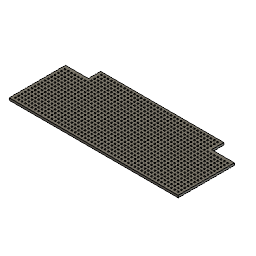
trunk mounting plate (Autodesk Fusion 360 design; units mm, degrees)
Autodesk Fusion 360 part; units mm, degrees
(part 1 of 2)
sketch "Sketch1" plane through (0, 0, 0) normal (0, 1, 0) x (1, 0, 0)
  line L0 (480, -195) -> (0, -195)
  line L1 (415, 0) -> (415, -35)
  line L2 (415, -35) -> (480, -35)
  line L3 (65, 0) -> (65, -35)
  line L4 (65, -35) -> (0, -35)
  line L5 (0, -195) -> (0, -35)
  line L6 (65, 0) -> (415, 0)
  line L7 (480, -35) -> (480, -195)
  circle A0 centre (9, -186) radius 2.25
  circle A1 centre (18.4286, -186) radius 2.25
  circle A2 centre (27.8571, -186) radius 2.25
  circle A3 centre (37.2857, -186) radius 2.25
  circle A4 centre (46.7143, -186) radius 2.25
  circle A5 centre (56.1429, -186) radius 2.25
  circle A6 centre (65.5714, -186) radius 2.25
  circle A7 centre (75, -186) radius 2.25
  circle A8 centre (84.4286, -186) radius 2.25
  circle A9 centre (93.8571, -186) radius 2.25
  circle A10 centre (103.2857, -186) radius 2.25
  circle A11 centre (112.7143, -186) radius 2.25
  circle A12 centre (122.1429, -186) radius 2.25
  circle A13 centre (131.5714, -186) radius 2.25
  circle A14 centre (141, -186) radius 2.25
  circle A15 centre (150.4286, -186) radius 2.25
  circle A16 centre (159.8571, -186) radius 2.25
  circle A17 centre (169.2857, -186) radius 2.25
  circle A18 centre (178.7143, -186) radius 2.25
  circle A19 centre (188.1429, -186) radius 2.25
  circle A20 centre (197.5714, -186) radius 2.25
  circle A21 centre (207, -186) radius 2.25
  circle A22 centre (216.4286, -186) radius 2.25
  circle A23 centre (225.8571, -186) radius 2.25
  circle A24 centre (235.2857, -186) radius 2.25
  circle A25 centre (244.7143, -186) radius 2.25
  circle A26 centre (254.1429, -186) radius 2.25
  circle A27 centre (263.5714, -186) radius 2.25
  circle A28 centre (273, -186) radius 2.25
  circle A29 centre (282.4286, -186) radius 2.25
  circle A30 centre (291.8571, -186) radius 2.25
  circle A31 centre (301.2857, -186) radius 2.25
  circle A32 centre (310.7143, -186) radius 2.25
  circle A33 centre (320.1429, -186) radius 2.25
  circle A34 centre (329.5714, -186) radius 2.25
  circle A35 centre (339, -186) radius 2.25
  circle A36 centre (348.4286, -186) radius 2.25
  circle A37 centre (357.8571, -186) radius 2.25
  circle A38 centre (367.2857, -186) radius 2.25
  circle A39 centre (376.7143, -186) radius 2.25
  circle A40 centre (386.1429, -186) radius 2.25
  circle A41 centre (395.5714, -186) radius 2.25
  circle A42 centre (405, -186) radius 2.25
  circle A43 centre (414.4286, -186) radius 2.25
  circle A44 centre (423.8571, -186) radius 2.25
  circle A45 centre (433.2857, -186) radius 2.25
  circle A46 centre (442.7143, -186) radius 2.25
  circle A47 centre (452.1429, -186) radius 2.25
  circle A48 centre (461.5714, -186) radius 2.25
  circle A49 centre (471, -186) radius 2.25
  circle A50 centre (9, -176.6421) radius 2.25
  circle A51 centre (18.4286, -176.6421) radius 2.25
  circle A52 centre (27.8571, -176.6421) radius 2.25
  circle A53 centre (37.2857, -176.6421) radius 2.25
  circle A54 centre (46.7143, -176.6421) radius 2.25
  circle A55 centre (56.1429, -176.6421) radius 2.25
  circle A56 centre (65.5714, -176.6421) radius 2.25
  circle A57 centre (75, -176.6421) radius 2.25
  circle A58 centre (84.4286, -176.6421) radius 2.25
  circle A59 centre (93.8571, -176.6421) radius 2.25
  circle A60 centre (103.2857, -176.6421) radius 2.25
  circle A61 centre (112.7143, -176.6421) radius 2.25
  circle A62 centre (122.1429, -176.6421) radius 2.25
  circle A63 centre (131.5714, -176.6421) radius 2.25
  circle A64 centre (141, -176.6421) radius 2.25
  circle A65 centre (150.4286, -176.6421) radius 2.25
  circle A66 centre (159.8571, -176.6421) radius 2.25
  circle A67 centre (169.2857, -176.6421) radius 2.25
  circle A68 centre (178.7143, -176.6421) radius 2.25
  circle A69 centre (188.1429, -176.6421) radius 2.25
  circle A70 centre (197.5714, -176.6421) radius 2.25
  circle A71 centre (207, -176.6421) radius 2.25
  circle A72 centre (216.4286, -176.6421) radius 2.25
  circle A73 centre (225.8571, -176.6421) radius 2.25
  circle A74 centre (235.2857, -176.6421) radius 2.25
  circle A75 centre (244.7143, -176.6421) radius 2.25
  circle A76 centre (254.1429, -176.6421) radius 2.25
  circle A77 centre (263.5714, -176.6421) radius 2.25
  circle A78 centre (273, -176.6421) radius 2.25
  circle A79 centre (282.4286, -176.6421) radius 2.25
  circle A80 centre (291.8571, -176.6421) radius 2.25
  circle A81 centre (301.2857, -176.6421) radius 2.25
  circle A82 centre (310.7143, -176.6421) radius 2.25
  circle A83 centre (320.1429, -176.6421) radius 2.25
  circle A84 centre (329.5714, -176.6421) radius 2.25
  circle A85 centre (339, -176.6421) radius 2.25
  circle A86 centre (348.4286, -176.6421) radius 2.25
  circle A87 centre (357.8571, -176.6421) radius 2.25
  circle A88 centre (367.2857, -176.6421) radius 2.25
  circle A89 centre (376.7143, -176.6421) radius 2.25
  circle A90 centre (386.1429, -176.6421) radius 2.25
  circle A91 centre (395.5714, -176.6421) radius 2.25
  circle A92 centre (405, -176.6421) radius 2.25
  circle A93 centre (414.4286, -176.6421) radius 2.25
  circle A94 centre (423.8571, -176.6421) radius 2.25
  circle A95 centre (433.2857, -176.6421) radius 2.25
  circle A96 centre (442.7143, -176.6421) radius 2.25
  circle A97 centre (452.1429, -176.6421) radius 2.25
  circle A98 centre (461.5714, -176.6421) radius 2.25
  circle A99 centre (471, -176.6421) radius 2.25
  circle A100 centre (9, -167.2842) radius 2.25
  circle A101 centre (18.4286, -167.2842) radius 2.25
  circle A102 centre (27.8571, -167.2842) radius 2.25
  circle A103 centre (37.2857, -167.2842) radius 2.25
  circle A104 centre (46.7143, -167.2842) radius 2.25
  circle A105 centre (56.1429, -167.2842) radius 2.25
  circle A106 centre (65.5714, -167.2842) radius 2.25
  circle A107 centre (75, -167.2842) radius 2.25
  circle A108 centre (84.4286, -167.2842) radius 2.25
  circle A109 centre (93.8571, -167.2842) radius 2.25
  circle A110 centre (103.2857, -167.2842) radius 2.25
  circle A111 centre (112.7143, -167.2842) radius 2.25
  circle A112 centre (122.1429, -167.2842) radius 2.25
  circle A113 centre (131.5714, -167.2842) radius 2.25
  circle A114 centre (141, -167.2842) radius 2.25
  circle A115 centre (150.4286, -167.2842) radius 2.25
  circle A116 centre (159.8571, -167.2842) radius 2.25
  circle A117 centre (169.2857, -167.2842) radius 2.25
  circle A118 centre (178.7143, -167.2842) radius 2.25
  circle A119 centre (188.1429, -167.2842) radius 2.25
  circle A120 centre (197.5714, -167.2842) radius 2.25
  circle A121 centre (207, -167.2842) radius 2.25
  circle A122 centre (216.4286, -167.2842) radius 2.25
  circle A123 centre (225.8571, -167.2842) radius 2.25
  circle A124 centre (235.2857, -167.2842) radius 2.25
  circle A125 centre (244.7143, -167.2842) radius 2.25
  circle A126 centre (254.1429, -167.2842) radius 2.25
  circle A127 centre (263.5714, -167.2842) radius 2.25
  circle A128 centre (273, -167.2842) radius 2.25
  circle A129 centre (282.4286, -167.2842) radius 2.25
  circle A130 centre (291.8571, -167.2842) radius 2.25
  circle A131 centre (301.2857, -167.2842) radius 2.25
  circle A132 centre (310.7143, -167.2842) radius 2.25
  circle A133 centre (320.1429, -167.2842) radius 2.25
  circle A134 centre (329.5714, -167.2842) radius 2.25
  circle A135 centre (339, -167.2842) radius 2.25
  circle A136 centre (348.4286, -167.2842) radius 2.25
  circle A137 centre (357.8571, -167.2842) radius 2.25
  circle A138 centre (367.2857, -167.2842) radius 2.25
  circle A139 centre (376.7143, -167.2842) radius 2.25
  circle A140 centre (386.1429, -167.2842) radius 2.25
  circle A141 centre (395.5714, -167.2842) radius 2.25
  circle A142 centre (405, -167.2842) radius 2.25
  circle A143 centre (414.4286, -167.2842) radius 2.25
  circle A144 centre (423.8571, -167.2842) radius 2.25
  circle A145 centre (433.2857, -167.2842) radius 2.25
  circle A146 centre (442.7143, -167.2842) radius 2.25
  circle A147 centre (452.1429, -167.2842) radius 2.25
  circle A148 centre (461.5714, -167.2842) radius 2.25
  circle A149 centre (471, -167.2842) radius 2.25
  circle A150 centre (9, -157.9263) radius 2.25
  circle A151 centre (18.4286, -157.9263) radius 2.25
  circle A152 centre (27.8571, -157.9263) radius 2.25
  circle A153 centre (37.2857, -157.9263) radius 2.25
  circle A154 centre (46.7143, -157.9263) radius 2.25
  circle A155 centre (56.1429, -157.9263) radius 2.25
  circle A156 centre (65.5714, -157.9263) radius 2.25
  circle A157 centre (75, -157.9263) radius 2.25
  circle A158 centre (84.4286, -157.9263) radius 2.25
  circle A159 centre (93.8571, -157.9263) radius 2.25
  circle A160 centre (103.2857, -157.9263) radius 2.25
  circle A161 centre (112.7143, -157.9263) radius 2.25
  circle A162 centre (122.1429, -157.9263) radius 2.25
  circle A163 centre (131.5714, -157.9263) radius 2.25
  circle A164 centre (141, -157.9263) radius 2.25
  circle A165 centre (150.4286, -157.9263) radius 2.25
  circle A166 centre (159.8571, -157.9263) radius 2.25
  circle A167 centre (169.2857, -157.9263) radius 2.25
  circle A168 centre (178.7143, -157.9263) radius 2.25
  circle A169 centre (188.1429, -157.9263) radius 2.25
  circle A170 centre (197.5714, -157.9263) radius 2.25
  circle A171 centre (207, -157.9263) radius 2.25
  circle A172 centre (216.4286, -157.9263) radius 2.25
  circle A173 centre (225.8571, -157.9263) radius 2.25
  circle A174 centre (235.2857, -157.9263) radius 2.25
  circle A175 centre (244.7143, -157.9263) radius 2.25
  circle A176 centre (254.1429, -157.9263) radius 2.25
  circle A177 centre (263.5714, -157.9263) radius 2.25
  circle A178 centre (273, -157.9263) radius 2.25
  circle A179 centre (282.4286, -157.9263) radius 2.25
  circle A180 centre (291.8571, -157.9263) radius 2.25
  circle A181 centre (301.2857, -157.9263) radius 2.25
  circle A182 centre (310.7143, -157.9263) radius 2.25
  circle A183 centre (320.1429, -157.9263) radius 2.25
  circle A184 centre (329.5714, -157.9263) radius 2.25
  circle A185 centre (339, -157.9263) radius 2.25
  circle A186 centre (348.4286, -157.9263) radius 2.25
  circle A187 centre (357.8571, -157.9263) radius 2.25
  circle A188 centre (367.2857, -157.9263) radius 2.25
  circle A189 centre (376.7143, -157.9263) radius 2.25
  circle A190 centre (386.1429, -157.9263) radius 2.25
  circle A191 centre (395.5714, -157.9263) radius 2.25
  circle A192 centre (405, -157.9263) radius 2.25
  circle A193 centre (414.4286, -157.9263) radius 2.25
  circle A194 centre (423.8571, -157.9263) radius 2.25
  circle A195 centre (433.2857, -157.9263) radius 2.25
  circle A196 centre (442.7143, -157.9263) radius 2.25
  circle A197 centre (452.1429, -157.9263) radius 2.25
  circle A198 centre (461.5714, -157.9263) radius 2.25
  circle A199 centre (471, -157.9263) radius 2.25
  circle A200 centre (9, -148.5684) radius 2.25
  circle A201 centre (18.4286, -148.5684) radius 2.25
  circle A202 centre (27.8571, -148.5684) radius 2.25
  circle A203 centre (37.2857, -148.5684) radius 2.25
  circle A204 centre (46.7143, -148.5684) radius 2.25
  circle A205 centre (56.1429, -148.5684) radius 2.25
  circle A206 centre (65.5714, -148.5684) radius 2.25
  circle A207 centre (75, -148.5684) radius 2.25
  circle A208 centre (84.4286, -148.5684) radius 2.25
  circle A209 centre (93.8571, -148.5684) radius 2.25
  circle A210 centre (103.2857, -148.5684) radius 2.25
  circle A211 centre (112.7143, -148.5684) radius 2.25
  circle A212 centre (122.1429, -148.5684) radius 2.25
  circle A213 centre (131.5714, -148.5684) radius 2.25
  circle A214 centre (141, -148.5684) radius 2.25
  circle A215 centre (150.4286, -148.5684) radius 2.25
  circle A216 centre (159.8571, -148.5684) radius 2.25
  circle A217 centre (169.2857, -148.5684) radius 2.25
  circle A218 centre (178.7143, -148.5684) radius 2.25
  circle A219 centre (188.1429, -148.5684) radius 2.25
  circle A220 centre (197.5714, -148.5684) radius 2.25
  circle A221 centre (207, -148.5684) radius 2.25
  circle A222 centre (216.4286, -148.5684) radius 2.25
  circle A223 centre (225.8571, -148.5684) radius 2.25
  circle A224 centre (235.2857, -148.5684) radius 2.25
  circle A225 centre (244.7143, -148.5684) radius 2.25
  circle A226 centre (254.1429, -148.5684) radius 2.25
  circle A227 centre (263.5714, -148.5684) radius 2.25
  circle A228 centre (273, -148.5684) radius 2.25
  circle A229 centre (282.4286, -148.5684) radius 2.25
  circle A230 centre (291.8571, -148.5684) radius 2.25
  circle A231 centre (301.2857, -148.5684) radius 2.25
  circle A232 centre (310.7143, -148.5684) radius 2.25
  circle A233 centre (320.1429, -148.5684) radius 2.25
  circle A234 centre (329.5714, -148.5684) radius 2.25
  circle A235 centre (339, -148.5684) radius 2.25
  circle A236 centre (348.4286, -148.5684) radius 2.25
  circle A237 centre (357.8571, -148.5684) radius 2.25
  circle A238 centre (367.2857, -148.5684) radius 2.25
  circle A239 centre (376.7143, -148.5684) radius 2.25
  circle A240 centre (386.1429, -148.5684) radius 2.25
  circle A241 centre (395.5714, -148.5684) radius 2.25
  circle A242 centre (405, -148.5684) radius 2.25
  circle A243 centre (414.4286, -148.5684) radius 2.25
  circle A244 centre (423.8571, -148.5684) radius 2.25
  circle A245 centre (433.2857, -148.5684) radius 2.25
  circle A246 centre (442.7143, -148.5684) radius 2.25
  circle A247 centre (452.1429, -148.5684) radius 2.25
  circle A248 centre (461.5714, -148.5684) radius 2.25
  circle A249 centre (471, -148.5684) radius 2.25
  circle A250 centre (9, -139.2105) radius 2.25
  circle A251 centre (18.4286, -139.2105) radius 2.25
  circle A252 centre (27.8571, -139.2105) radius 2.25
  circle A253 centre (37.2857, -139.2105) radius 2.25
  circle A254 centre (46.7143, -139.2105) radius 2.25
  circle A255 centre (56.1429, -139.2105) radius 2.25
  circle A256 centre (65.5714, -139.2105) radius 2.25
  circle A257 centre (75, -139.2105) radius 2.25
  circle A258 centre (84.4286, -139.2105) radius 2.25
  circle A259 centre (93.8571, -139.2105) radius 2.25
  circle A260 centre (103.2857, -139.2105) radius 2.25
  circle A261 centre (112.7143, -139.2105) radius 2.25
  circle A262 centre (122.1429, -139.2105) radius 2.25
  circle A263 centre (131.5714, -139.2105) radius 2.25
  circle A264 centre (141, -139.2105) radius 2.25
  circle A265 centre (150.4286, -139.2105) radius 2.25
  circle A266 centre (159.8571, -139.2105) radius 2.25
  circle A267 centre (169.2857, -139.2105) radius 2.25
  circle A268 centre (178.7143, -139.2105) radius 2.25
  circle A269 centre (188.1429, -139.2105) radius 2.25
  circle A270 centre (197.5714, -139.2105) radius 2.25
  circle A271 centre (207, -139.2105) radius 2.25
  circle A272 centre (216.4286, -139.2105) radius 2.25
  circle A273 centre (225.8571, -139.2105) radius 2.25
  circle A274 centre (235.2857, -139.2105) radius 2.25
  circle A275 centre (244.7143, -139.2105) radius 2.25
  circle A276 centre (254.1429, -139.2105) radius 2.25
  circle A277 centre (263.5714, -139.2105) radius 2.25
  circle A278 centre (273, -139.2105) radius 2.25
  circle A279 centre (282.4286, -139.2105) radius 2.25
  circle A280 centre (291.8571, -139.2105) radius 2.25
  circle A281 centre (301.2857, -139.2105) radius 2.25
  circle A282 centre (310.7143, -139.2105) radius 2.25
  circle A283 centre (320.1429, -139.2105) radius 2.25
  circle A284 centre (329.5714, -139.2105) radius 2.25
  circle A285 centre (339, -139.2105) radius 2.25
  circle A286 centre (348.4286, -139.2105) radius 2.25
  circle A287 centre (357.8571, -139.2105) radius 2.25
  circle A288 centre (367.2857, -139.2105) radius 2.25
  circle A289 centre (376.7143, -139.2105) radius 2.25
  circle A290 centre (386.1429, -139.2105) radius 2.25
  circle A291 centre (395.5714, -139.2105) radius 2.25
  circle A292 centre (405, -139.2105) radius 2.25
  circle A293 centre (414.4286, -139.2105) radius 2.25
  circle A294 centre (423.8571, -139.2105) radius 2.25
  circle A295 centre (433.2857, -139.2105) radius 2.25
  circle A296 centre (442.7143, -139.2105) radius 2.25
  circle A297 centre (452.1429, -139.2105) radius 2.25
  circle A298 centre (461.5714, -139.2105) radius 2.25
  circle A299 centre (471, -139.2105) radius 2.25
  circle A300 centre (9, -129.8526) radius 2.25
  circle A301 centre (18.4286, -129.8526) radius 2.25
  circle A302 centre (27.8571, -129.8526) radius 2.25
  circle A303 centre (37.2857, -129.8526) radius 2.25
  circle A304 centre (46.7143, -129.8526) radius 2.25
  circle A305 centre (56.1429, -129.8526) radius 2.25
  circle A306 centre (65.5714, -129.8526) radius 2.25
  circle A307 centre (75, -129.8526) radius 2.25
  circle A308 centre (84.4286, -129.8526) radius 2.25
  circle A309 centre (93.8571, -129.8526) radius 2.25
  circle A310 centre (103.2857, -129.8526) radius 2.25
  circle A311 centre (112.7143, -129.8526) radius 2.25
  circle A312 centre (122.1429, -129.8526) radius 2.25
  circle A313 centre (131.5714, -129.8526) radius 2.25
  circle A314 centre (141, -129.8526) radius 2.25
  circle A315 centre (150.4286, -129.8526) radius 2.25
  circle A316 centre (159.8571, -129.8526) radius 2.25
  circle A317 centre (169.2857, -129.8526) radius 2.25
  circle A318 centre (178.7143, -129.8526) radius 2.25
  circle A319 centre (188.1429, -129.8526) radius 2.25
  circle A320 centre (197.5714, -129.8526) radius 2.25
  circle A321 centre (207, -129.8526) radius 2.25
  circle A322 centre (216.4286, -129.8526) radius 2.25
  circle A323 centre (225.8571, -129.8526) radius 2.25
  circle A324 centre (235.2857, -129.8526) radius 2.25
  circle A325 centre (244.7143, -129.8526) radius 2.25
  circle A326 centre (254.1429, -129.8526) radius 2.25
  circle A327 centre (263.5714, -129.8526) radius 2.25
  circle A328 centre (273, -129.8526) radius 2.25
  circle A329 centre (282.4286, -129.8526) radius 2.25
  circle A330 centre (291.8571, -129.8526) radius 2.25
  circle A331 centre (301.2857, -129.8526) radius 2.25
  circle A332 centre (310.7143, -129.8526) radius 2.25
  circle A333 centre (320.1429, -129.8526) radius 2.25
  circle A334 centre (329.5714, -129.8526) radius 2.25
  circle A335 centre (339, -129.8526) radius 2.25
  circle A336 centre (348.4286, -129.8526) radius 2.25
  circle A337 centre (357.8571, -129.8526) radius 2.25
  circle A338 centre (367.2857, -129.8526) radius 2.25
  circle A339 centre (376.7143, -129.8526) radius 2.25
  circle A340 centre (386.1429, -129.8526) radius 2.25
  circle A341 centre (395.5714, -129.8526) radius 2.25
  circle A342 centre (405, -129.8526) radius 2.25
  circle A343 centre (414.4286, -129.8526) radius 2.25
  circle A344 centre (423.8571, -129.8526) radius 2.25
  circle A345 centre (433.2857, -129.8526) radius 2.25
  circle A346 centre (442.7143, -129.8526) radius 2.25
  circle A347 centre (452.1429, -129.8526) radius 2.25
  circle A348 centre (461.5714, -129.8526) radius 2.25
  circle A349 centre (471, -129.8526) radius 2.25
  circle A350 centre (9, -120.4947) radius 2.25
  circle A351 centre (18.4286, -120.4947) radius 2.25
  circle A352 centre (27.8571, -120.4947) radius 2.25
  circle A353 centre (37.2857, -120.4947) radius 2.25
  circle A354 centre (46.7143, -120.4947) radius 2.25
  circle A355 centre (56.1429, -120.4947) radius 2.25
  circle A356 centre (65.5714, -120.4947) radius 2.25
  circle A357 centre (75, -120.4947) radius 2.25
  circle A358 centre (84.4286, -120.4947) radius 2.25
  circle A359 centre (93.8571, -120.4947) radius 2.25
  circle A360 centre (103.2857, -120.4947) radius 2.25
  circle A361 centre (112.7143, -120.4947) radius 2.25
  circle A362 centre (122.1429, -120.4947) radius 2.25
  circle A363 centre (131.5714, -120.4947) radius 2.25
  circle A364 centre (141, -120.4947) radius 2.25
  circle A365 centre (150.4286, -120.4947) radius 2.25
  circle A366 centre (159.8571, -120.4947) radius 2.25
  circle A367 centre (169.2857, -120.4947) radius 2.25
  circle A368 centre (178.7143, -120.4947) radius 2.25
  circle A369 centre (188.1429, -120.4947) radius 2.25
  circle A370 centre (197.5714, -120.4947) radius 2.25
  circle A371 centre (207, -120.4947) radius 2.25
  circle A372 centre (216.4286, -120.4947) radius 2.25
  circle A373 centre (225.8571, -120.4947) radius 2.25
  circle A374 centre (235.2857, -120.4947) radius 2.25
  circle A375 centre (244.7143, -120.4947) radius 2.25
  circle A376 centre (254.1429, -120.4947) radius 2.25
  circle A377 centre (263.5714, -120.4947) radius 2.25
  circle A378 centre (273, -120.4947) radius 2.25
  circle A379 centre (282.4286, -120.4947) radius 2.25
  circle A380 centre (291.8571, -120.4947) radius 2.25
  circle A381 centre (301.2857, -120.4947) radius 2.25
  circle A382 centre (310.7143, -120.4947) radius 2.25
  circle A383 centre (320.1429, -120.4947) radius 2.25
  circle A384 centre (329.5714, -120.4947) radius 2.25
  circle A385 centre (339, -120.4947) radius 2.25
  circle A386 centre (348.4286, -120.4947) radius 2.25
  circle A387 centre (357.8571, -120.4947) radius 2.25
  circle A388 centre (367.2857, -120.4947) radius 2.25
  circle A389 centre (376.7143, -120.4947) radius 2.25
  circle A390 centre (386.1429, -120.4947) radius 2.25
  circle A391 centre (395.5714, -120.4947) radius 2.25
  circle A392 centre (405, -120.4947) radius 2.25
  circle A393 centre (414.4286, -120.4947) radius 2.25
  circle A394 centre (423.8571, -120.4947) radius 2.25
  circle A395 centre (433.2857, -120.4947) radius 2.25
  circle A396 centre (442.7143, -120.4947) radius 2.25
  circle A397 centre (452.1429, -120.4947) radius 2.25
  circle A398 centre (461.5714, -120.4947) radius 2.25
  circle A399 centre (471, -120.4947) radius 2.25
  circle A400 centre (9, -111.1368) radius 2.25
  circle A401 centre (18.4286, -111.1368) radius 2.25
  circle A402 centre (27.8571, -111.1368) radius 2.25
  circle A403 centre (37.2857, -111.1368) radius 2.25
  circle A404 centre (46.7143, -111.1368) radius 2.25
  circle A405 centre (56.1429, -111.1368) radius 2.25
  circle A406 centre (65.5714, -111.1368) radius 2.25
  circle A407 centre (75, -111.1368) radius 2.25
  circle A408 centre (84.4286, -111.1368) radius 2.25
  circle A409 centre (93.8571, -111.1368) radius 2.25
  circle A410 centre (103.2857, -111.1368) radius 2.25
  circle A411 centre (112.7143, -111.1368) radius 2.25
  circle A412 centre (122.1429, -111.1368) radius 2.25
  circle A413 centre (131.5714, -111.1368) radius 2.25
  circle A414 centre (141, -111.1368) radius 2.25
  circle A415 centre (150.4286, -111.1368) radius 2.25
  circle A416 centre (159.8571, -111.1368) radius 2.25
  circle A417 centre (169.2857, -111.1368) radius 2.25
  circle A418 centre (178.7143, -111.1368) radius 2.25
  circle A419 centre (188.1429, -111.1368) radius 2.25
  circle A420 centre (197.5714, -111.1368) radius 2.25
  circle A421 centre (207, -111.1368) radius 2.25
  circle A422 centre (216.4286, -111.1368) radius 2.25
  circle A423 centre (225.8571, -111.1368) radius 2.25
  circle A424 centre (235.2857, -111.1368) radius 2.25
  circle A425 centre (244.7143, -111.1368) radius 2.25
  circle A426 centre (254.1429, -111.1368) radius 2.25
  circle A427 centre (263.5714, -111.1368) radius 2.25
  circle A428 centre (273, -111.1368) radius 2.25
  circle A429 centre (282.4286, -111.1368) radius 2.25
  circle A430 centre (291.8571, -111.1368) radius 2.25
  circle A431 centre (301.2857, -111.1368) radius 2.25
  circle A432 centre (310.7143, -111.1368) radius 2.25
  circle A433 centre (320.1429, -111.1368) radius 2.25
  circle A434 centre (329.5714, -111.1368) radius 2.25
  circle A435 centre (339, -111.1368) radius 2.25
  circle A436 centre (348.4286, -111.1368) radius 2.25
  circle A437 centre (357.8571, -111.1368) radius 2.25
  circle A438 centre (367.2857, -111.1368) radius 2.25
  circle A439 centre (376.7143, -111.1368) radius 2.25
  circle A440 centre (386.1429, -111.1368) radius 2.25
  circle A441 centre (395.5714, -111.1368) radius 2.25
  circle A442 centre (405, -111.1368) radius 2.25
  circle A443 centre (414.4286, -111.1368) radius 2.25
  circle A444 centre (423.8571, -111.1368) radius 2.25
  circle A445 centre (433.2857, -111.1368) radius 2.25
  circle A446 centre (442.7143, -111.1368) radius 2.25
  circle A447 centre (452.1429, -111.1368) radius 2.25
  circle A448 centre (461.5714, -111.1368) radius 2.25
  circle A449 centre (471, -111.1368) radius 2.25
  circle A450 centre (9, -101.7789) radius 2.25
  circle A451 centre (18.4286, -101.7789) radius 2.25
  circle A452 centre (27.8571, -101.7789) radius 2.25
  circle A453 centre (37.2857, -101.7789) radius 2.25
  circle A454 centre (46.7143, -101.7789) radius 2.25
  circle A455 centre (56.1429, -101.7789) radius 2.25
  circle A456 centre (65.5714, -101.7789) radius 2.25
  circle A457 centre (75, -101.7789) radius 2.25
  circle A458 centre (84.4286, -101.7789) radius 2.25
  circle A459 centre (93.8571, -101.7789) radius 2.25
  circle A460 centre (103.2857, -101.7789) radius 2.25
  circle A461 centre (112.7143, -101.7789) radius 2.25
  circle A462 centre (122.1429, -101.7789) radius 2.25
  circle A463 centre (131.5714, -101.7789) radius 2.25
  circle A464 centre (141, -101.7789) radius 2.25
  circle A465 centre (150.4286, -101.7789) radius 2.25
  circle A466 centre (159.8571, -101.7789) radius 2.25
  circle A467 centre (169.2857, -101.7789) radius 2.25
  circle A468 centre (178.7143, -101.7789) radius 2.25
  circle A469 centre (188.1429, -101.7789) radius 2.25
  circle A470 centre (197.5714, -101.7789) radius 2.25
  circle A471 centre (207, -101.7789) radius 2.25
  circle A472 centre (216.4286, -101.7789) radius 2.25
  circle A473 centre (225.8571, -101.7789) radius 2.25
  circle A474 centre (235.2857, -101.7789) radius 2.25
  circle A475 centre (244.7143, -101.7789) radius 2.25
  circle A476 centre (254.1429, -101.7789) radius 2.25
  circle A477 centre (263.5714, -101.7789) radius 2.25
  circle A478 centre (273, -101.7789) radius 2.25
  circle A479 centre (282.4286, -101.7789) radius 2.25
  circle A480 centre (291.8571, -101.7789) radius 2.25
  circle A481 centre (301.2857, -101.7789) radius 2.25
  circle A482 centre (310.7143, -101.7789) radius 2.25
  circle A483 centre (320.1429, -101.7789) radius 2.25
  circle A484 centre (329.5714, -101.7789) radius 2.25
  circle A485 centre (339, -101.7789) radius 2.25
  circle A486 centre (348.4286, -101.7789) radius 2.25
  circle A487 centre (357.8571, -101.7789) radius 2.25
  circle A488 centre (367.2857, -101.7789) radius 2.25
  circle A489 centre (376.7143, -101.7789) radius 2.25
  circle A490 centre (386.1429, -101.7789) radius 2.25
  circle A491 centre (395.5714, -101.7789) radius 2.25
  circle A492 centre (405, -101.7789) radius 2.25
  circle A493 centre (414.4286, -101.7789) radius 2.25
  circle A494 centre (423.8571, -101.7789) radius 2.25
  circle A495 centre (433.2857, -101.7789) radius 2.25
  circle A496 centre (442.7143, -101.7789) radius 2.25
  circle A497 centre (452.1429, -101.7789) radius 2.25
  circle A498 centre (461.5714, -101.7789) radius 2.25
  circle A499 centre (471, -101.7789) radius 2.25
  circle A500 centre (9, -92.4211) radius 2.25
  circle A501 centre (18.4286, -92.4211) radius 2.25
  circle A502 centre (27.8571, -92.4211) radius 2.25
  circle A503 centre (37.2857, -92.4211) radius 2.25
  circle A504 centre (46.7143, -92.4211) radius 2.25
  circle A505 centre (56.1429, -92.4211) radius 2.25
  circle A506 centre (65.5714, -92.4211) radius 2.25
  circle A507 centre (75, -92.4211) radius 2.25
  circle A508 centre (84.4286, -92.4211) radius 2.25
  circle A509 centre (93.8571, -92.4211) radius 2.25
  circle A510 centre (103.2857, -92.4211) radius 2.25
  circle A511 centre (112.7143, -92.4211) radius 2.25
  circle A512 centre (122.1429, -92.4211) radius 2.25
  circle A513 centre (131.5714, -92.4211) radius 2.25
  circle A514 centre (141, -92.4211) radius 2.25
  circle A515 centre (150.4286, -92.4211) radius 2.25
  circle A516 centre (159.8571, -92.4211) radius 2.25
  circle A517 centre (169.2857, -92.4211) radius 2.25
  circle A518 centre (178.7143, -92.4211) radius 2.25
  circle A519 centre (188.1429, -92.4211) radius 2.25
  circle A520 centre (197.5714, -92.4211) radius 2.25
  circle A521 centre (207, -92.4211) radius 2.25
  circle A522 centre (216.4286, -92.4211) radius 2.25
  circle A523 centre (225.8571, -92.4211) radius 2.25
  circle A524 centre (235.2857, -92.4211) radius 2.25
  circle A525 centre (244.7143, -92.4211) radius 2.25
  circle A526 centre (254.1429, -92.4211) radius 2.25
  circle A527 centre (263.5714, -92.4211) radius 2.25
  circle A528 centre (273, -92.4211) radius 2.25
  circle A529 centre (282.4286, -92.4211) radius 2.25
  circle A530 centre (291.8571, -92.4211) radius 2.25
  circle A531 centre (301.2857, -92.4211) radius 2.25
  circle A532 centre (310.7143, -92.4211) radius 2.25
  circle A533 centre (320.1429, -92.4211) radius 2.25
  circle A534 centre (329.5714, -92.4211) radius 2.25
  circle A535 centre (339, -92.4211) radius 2.25
  circle A536 centre (348.4286, -92.4211) radius 2.25
  circle A537 centre (357.8571, -92.4211) radius 2.25
  circle A538 centre (367.2857, -92.4211) radius 2.25
  circle A539 centre (376.7143, -92.4211) radius 2.25
  circle A540 centre (386.1429, -92.4211) radius 2.25
  circle A541 centre (395.5714, -92.4211) radius 2.25
  circle A542 centre (405, -92.4211) radius 2.25
  circle A543 centre (414.4286, -92.4211) radius 2.25
  circle A544 centre (423.8571, -92.4211) radius 2.25
  circle A545 centre (433.2857, -92.4211) radius 2.25
  circle A546 centre (442.7143, -92.4211) radius 2.25
  circle A547 centre (452.1429, -92.4211) radius 2.25
  circle A548 centre (461.5714, -92.4211) radius 2.25
  circle A549 centre (471, -92.4211) radius 2.25
  circle A550 centre (9, -83.0632) radius 2.25
  circle A551 centre (18.4286, -83.0632) radius 2.25
  circle A552 centre (27.8571, -83.0632) radius 2.25
  circle A553 centre (37.2857, -83.0632) radius 2.25
  circle A554 centre (46.7143, -83.0632) radius 2.25
  circle A555 centre (56.1429, -83.0632) radius 2.25
  circle A556 centre (65.5714, -83.0632) radius 2.25
  circle A557 centre (75, -83.0632) radius 2.25
  circle A558 centre (84.4286, -83.0632) radius 2.25
  circle A559 centre (93.8571, -83.0632) radius 2.25
  circle A560 centre (103.2857, -83.0632) radius 2.25
  circle A561 centre (112.7143, -83.0632) radius 2.25
  circle A562 centre (122.1429, -83.0632) radius 2.25
  circle A563 centre (131.5714, -83.0632) radius 2.25
  circle A564 centre (141, -83.0632) radius 2.25
  circle A565 centre (150.4286, -83.0632) radius 2.25
  circle A566 centre (159.8571, -83.0632) radius 2.25
  circle A567 centre (169.2857, -83.0632) radius 2.25
  circle A568 centre (178.7143, -83.0632) radius 2.25
  circle A569 centre (188.1429, -83.0632) radius 2.25
  circle A570 centre (197.5714, -83.0632) radius 2.25
  circle A571 centre (207, -83.0632) radius 2.25
  circle A572 centre (216.4286, -83.0632) radius 2.25
  circle A573 centre (225.8571, -83.0632) radius 2.25
  circle A574 centre (235.2857, -83.0632) radius 2.25
  circle A575 centre (244.7143, -83.0632) radius 2.25
  circle A576 centre (254.1429, -83.0632) radius 2.25
  circle A577 centre (263.5714, -83.0632) radius 2.25
  circle A578 centre (273, -83.0632) radius 2.25
  circle A579 centre (282.4286, -83.0632) radius 2.25
  circle A580 centre (291.8571, -83.0632) radius 2.25
  circle A581 centre (301.2857, -83.0632) radius 2.25
  circle A582 centre (310.7143, -83.0632) radius 2.25
  circle A583 centre (320.1429, -83.0632) radius 2.25
  circle A584 centre (329.5714, -83.0632) radius 2.25
  circle A585 centre (339, -83.0632) radius 2.25
  circle A586 centre (348.4286, -83.0632) radius 2.25
  circle A587 centre (357.8571, -83.0632) radius 2.25
  circle A588 centre (367.2857, -83.0632) radius 2.25
  circle A589 centre (376.7143, -83.0632) radius 2.25
  circle A590 centre (386.1429, -83.0632) radius 2.25
  circle A591 centre (395.5714, -83.0632) radius 2.25
  circle A592 centre (405, -83.0632) radius 2.25
  circle A593 centre (414.4286, -83.0632) radius 2.25
  circle A594 centre (423.8571, -83.0632) radius 2.25
  circle A595 centre (433.2857, -83.0632) radius 2.25
  circle A596 centre (442.7143, -83.0632) radius 2.25
  circle A597 centre (452.1429, -83.0632) radius 2.25
  circle A598 centre (461.5714, -83.0632) radius 2.25
  circle A599 centre (471, -83.0632) radius 2.25
  circle A600 centre (9, -73.7053) radius 2.25
  circle A601 centre (18.4286, -73.7053) radius 2.25
  circle A602 centre (27.8571, -73.7053) radius 2.25
  circle A603 centre (37.2857, -73.7053) radius 2.25
  circle A604 centre (46.7143, -73.7053) radius 2.25
  circle A605 centre (56.1429, -73.7053) radius 2.25
  circle A606 centre (65.5714, -73.7053) radius 2.25
  circle A607 centre (75, -73.7053) radius 2.25
  circle A608 centre (84.4286, -73.7053) radius 2.25
  circle A609 centre (93.8571, -73.7053) radius 2.25
  circle A610 centre (103.2857, -73.7053) radius 2.25
  circle A611 centre (112.7143, -73.7053) radius 2.25
  circle A612 centre (122.1429, -73.7053) radius 2.25
  circle A613 centre (131.5714, -73.7053) radius 2.25
  circle A614 centre (141, -73.7053) radius 2.25
  circle A615 centre (150.4286, -73.7053) radius 2.25
  circle A616 centre (159.8571, -73.7053) radius 2.25
  circle A617 centre (169.2857, -73.7053) radius 2.25
  circle A618 centre (178.7143, -73.7053) radius 2.25
  circle A619 centre (188.1429, -73.7053) radius 2.25
  circle A620 centre (197.5714, -73.7053) radius 2.25
  circle A621 centre (207, -73.7053) radius 2.25
  circle A622 centre (216.4286, -73.7053) radius 2.25
  circle A623 centre (225.8571, -73.7053) radius 2.25
  circle A624 centre (235.2857, -73.7053) radius 2.25
  circle A625 centre (244.7143, -73.7053) radius 2.25
  circle A626 centre (254.1429, -73.7053) radius 2.25
  circle A627 centre (263.5714, -73.7053) radius 2.25
  circle A628 centre (273, -73.7053) radius 2.25
  circle A629 centre (282.4286, -73.7053) radius 2.25
  circle A630 centre (291.8571, -73.7053) radius 2.25
  circle A631 centre (301.2857, -73.7053) radius 2.25
  circle A632 centre (310.7143, -73.7053) radius 2.25
  circle A633 centre (320.1429, -73.7053) radius 2.25
  circle A634 centre (329.5714, -73.7053) radius 2.25
  circle A635 centre (339, -73.7053) radius 2.25
  circle A636 centre (348.4286, -73.7053) radius 2.25
  circle A637 centre (357.8571, -73.7053) radius 2.25
  circle A638 centre (367.2857, -73.7053) radius 2.25
  circle A639 centre (376.7143, -73.7053) radius 2.25
  circle A640 centre (386.1429, -73.7053) radius 2.25
  circle A641 centre (395.5714, -73.7053) radius 2.25
  circle A642 centre (405, -73.7053) radius 2.25
  circle A643 centre (414.4286, -73.7053) radius 2.25
  circle A644 centre (423.8571, -73.7053) radius 2.25
  circle A645 centre (433.2857, -73.7053) radius 2.25
  circle A646 centre (442.7143, -73.7053) radius 2.25
  circle A647 centre (452.1429, -73.7053) radius 2.25
  circle A648 centre (461.5714, -73.7053) radius 2.25
  circle A649 centre (471, -73.7053) radius 2.25
  circle A650 centre (9, -64.3474) radius 2.25
  circle A651 centre (18.4286, -64.3474) radius 2.25
  circle A652 centre (27.8571, -64.3474) radius 2.25
  circle A653 centre (37.2857, -64.3474) radius 2.25
  circle A654 centre (46.7143, -64.3474) radius 2.25
  circle A655 centre (56.1429, -64.3474) radius 2.25
  circle A656 centre (65.5714, -64.3474) radius 2.25
  circle A657 centre (75, -64.3474) radius 2.25
  circle A658 centre (84.4286, -64.3474) radius 2.25
  circle A659 centre (93.8571, -64.3474) radius 2.25
  circle A660 centre (103.2857, -64.3474) radius 2.25
  circle A661 centre (112.7143, -64.3474) radius 2.25
  circle A662 centre (122.1429, -64.3474) radius 2.25
  circle A663 centre (131.5714, -64.3474) radius 2.25
  circle A664 centre (141, -64.3474) radius 2.25
  circle A665 centre (150.4286, -64.3474) radius 2.25
  circle A666 centre (159.8571, -64.3474) radius 2.25
  circle A667 centre (169.2857, -64.3474) radius 2.25
  circle A668 centre (178.7143, -64.3474) radius 2.25
  circle A669 centre (188.1429, -64.3474) radius 2.25
  circle A670 centre (197.5714, -64.3474) radius 2.25
  circle A671 centre (207, -64.3474) radius 2.25
  circle A672 centre (216.4286, -64.3474) radius 2.25
  circle A673 centre (225.8571, -64.3474) radius 2.25
  circle A674 centre (235.2857, -64.3474) radius 2.25
  circle A675 centre (244.7143, -64.3474) radius 2.25
  circle A676 centre (254.1429, -64.3474) radius 2.25
  circle A677 centre (263.5714, -64.3474) radius 2.25
  circle A678 centre (273, -64.3474) radius 2.25
  circle A679 centre (282.4286, -64.3474) radius 2.25
  circle A680 centre (291.8571, -64.3474) radius 2.25
  circle A681 centre (301.2857, -64.3474) radius 2.25
  circle A682 centre (310.7143, -64.3474) radius 2.25
  circle A683 centre (320.1429, -64.3474) radius 2.25
  circle A684 centre (329.5714, -64.3474) radius 2.25
  circle A685 centre (339, -64.3474) radius 2.25
  circle A686 centre (348.4286, -64.3474) radius 2.25
  circle A687 centre (357.8571, -64.3474) radius 2.25
  circle A688 centre (367.2857, -64.3474) radius 2.25
  circle A689 centre (376.7143, -64.3474) radius 2.25
  circle A690 centre (386.1429, -64.3474) radius 2.25
  circle A691 centre (395.5714, -64.3474) radius 2.25
  circle A692 centre (405, -64.3474) radius 2.25
  circle A693 centre (414.4286, -64.3474) radius 2.25
  circle A694 centre (423.8571, -64.3474) radius 2.25
  circle A695 centre (433.2857, -64.3474) radius 2.25
  circle A696 centre (442.7143, -64.3474) radius 2.25
  circle A697 centre (452.1429, -64.3474) radius 2.25
  circle A698 centre (461.5714, -64.3474) radius 2.25
  circle A699 centre (471, -64.3474) radius 2.25
  circle A700 centre (9, -54.9895) radius 2.25
  circle A701 centre (18.4286, -54.9895) radius 2.25
  circle A702 centre (27.8571, -54.9895) radius 2.25
  circle A703 centre (37.2857, -54.9895) radius 2.25
  circle A704 centre (46.7143, -54.9895) radius 2.25
  circle A705 centre (56.1429, -54.9895) radius 2.25
  circle A706 centre (65.5714, -54.9895) radius 2.25
  circle A707 centre (75, -54.9895) radius 2.25
  circle A708 centre (84.4286, -54.9895) radius 2.25
  circle A709 centre (93.8571, -54.9895) radius 2.25
  circle A710 centre (103.2857, -54.9895) radius 2.25
  circle A711 centre (112.7143, -54.9895) radius 2.25
  circle A712 centre (122.1429, -54.9895) radius 2.25
  circle A713 centre (131.5714, -54.9895) radius 2.25
  circle A714 centre (141, -54.9895) radius 2.25
  circle A715 centre (150.4286, -54.9895) radius 2.25
  circle A716 centre (159.8571, -54.9895) radius 2.25
  circle A717 centre (169.2857, -54.9895) radius 2.25
  circle A718 centre (178.7143, -54.9895) radius 2.25
  circle A719 centre (188.1429, -54.9895) radius 2.25
  circle A720 centre (197.5714, -54.9895) radius 2.25
  circle A721 centre (207, -54.9895) radius 2.25
  circle A722 centre (216.4286, -54.9895) radius 2.25
  circle A723 centre (225.8571, -54.9895) radius 2.25
  circle A724 centre (235.2857, -54.9895) radius 2.25
  circle A725 centre (244.7143, -54.9895) radius 2.25
  circle A726 centre (254.1429, -54.9895) radius 2.25
  circle A727 centre (263.5714, -54.9895) radius 2.25
  circle A728 centre (273, -54.9895) radius 2.25
  circle A729 centre (282.4286, -54.9895) radius 2.25
  circle A730 centre (291.8571, -54.9895) radius 2.25
  circle A731 centre (301.2857, -54.9895) radius 2.25
  circle A732 centre (310.7143, -54.9895) radius 2.25
  circle A733 centre (320.1429, -54.9895) radius 2.25
  circle A734 centre (329.5714, -54.9895) radius 2.25
  circle A735 centre (339, -54.9895) radius 2.25
  circle A736 centre (348.4286, -54.9895) radius 2.25
  circle A737 centre (357.8571, -54.9895) radius 2.25
  circle A738 centre (367.2857, -54.9895) radius 2.25
  circle A739 centre (376.7143, -54.9895) radius 2.25
  circle A740 centre (386.1429, -54.9895) radius 2.25
  circle A741 centre (395.5714, -54.9895) radius 2.25
  circle A742 centre (405, -54.9895) radius 2.25
  circle A743 centre (414.4286, -54.9895) radius 2.25
  circle A744 centre (423.8571, -54.9895) radius 2.25
  circle A745 centre (433.2857, -54.9895) radius 2.25
  circle A746 centre (442.7143, -54.9895) radius 2.25
  circle A747 centre (452.1429, -54.9895) radius 2.25
  circle A748 centre (461.5714, -54.9895) radius 2.25
  circle A749 centre (471, -54.9895) radius 2.25
  circle A750 centre (9, -45.6316) radius 2.25
  circle A751 centre (18.4286, -45.6316) radius 2.25
  circle A752 centre (27.8571, -45.6316) radius 2.25
  circle A753 centre (37.2857, -45.6316) radius 2.25
  circle A754 centre (46.7143, -45.6316) radius 2.25
  circle A755 centre (56.1429, -45.6316) radius 2.25
  circle A756 centre (65.5714, -45.6316) radius 2.25
  circle A757 centre (75, -45.6316) radius 2.25
  circle A758 centre (84.4286, -45.6316) radius 2.25
  circle A759 centre (93.8571, -45.6316) radius 2.25
  circle A760 centre (103.2857, -45.6316) radius 2.25
  circle A761 centre (112.7143, -45.6316) radius 2.25
  circle A762 centre (122.1429, -45.6316) radius 2.25
  circle A763 centre (131.5714, -45.6316) radius 2.25
  circle A764 centre (141, -45.6316) radius 2.25
  circle A765 centre (150.4286, -45.6316) radius 2.25
  circle A766 centre (159.8571, -45.6316) radius 2.25
  circle A767 centre (169.2857, -45.6316) radius 2.25
  circle A768 centre (178.7143, -45.6316) radius 2.25
  circle A769 centre (188.1429, -45.6316) radius 2.25
  circle A770 centre (197.5714, -45.6316) radius 2.25
  circle A771 centre (207, -45.6316) radius 2.25
  circle A772 centre (216.4286, -45.6316) radius 2.25
  circle A773 centre (225.8571, -45.6316) radius 2.25
  circle A774 centre (235.2857, -45.6316) radius 2.25
  circle A775 centre (244.7143, -45.6316) radius 2.25
  circle A776 centre (254.1429, -45.6316) radius 2.25
  circle A777 centre (263.5714, -45.6316) radius 2.25
  circle A778 centre (273, -45.6316) radius 2.25
  circle A779 centre (282.4286, -45.6316) radius 2.25
  circle A780 centre (291.8571, -45.6316) radius 2.25
  circle A781 centre (301.2857, -45.6316) radius 2.25
  circle A782 centre (310.7143, -45.6316) radius 2.25
  circle A783 centre (320.1429, -45.6316) radius 2.25
  circle A784 centre (329.5714, -45.6316) radius 2.25
  circle A785 centre (339, -45.6316) radius 2.25
  circle A786 centre (348.4286, -45.6316) radius 2.25
  circle A787 centre (357.8571, -45.6316) radius 2.25
  circle A788 centre (367.2857, -45.6316) radius 2.25
  circle A789 centre (376.7143, -45.6316) radius 2.25
  circle A790 centre (386.1429, -45.6316) radius 2.25
  circle A791 centre (395.5714, -45.6316) radius 2.25
  circle A792 centre (405, -45.6316) radius 2.25
  circle A793 centre (414.4286, -45.6316) radius 2.25
  circle A794 centre (423.8571, -45.6316) radius 2.25
  circle A795 centre (433.2857, -45.6316) radius 2.25
  circle A796 centre (442.7143, -45.6316) radius 2.25
  circle A797 centre (452.1429, -45.6316) radius 2.25
  circle A798 centre (461.5714, -45.6316) radius 2.25
  circle A799 centre (471, -45.6316) radius 2.25
  circle A800 centre (75, -36.2737) radius 2.25
  circle A801 centre (84.4286, -36.2737) radius 2.25
  circle A802 centre (93.8571, -36.2737) radius 2.25
  circle A803 centre (103.2857, -36.2737) radius 2.25
  circle A804 centre (112.7143, -36.2737) radius 2.25
  circle A805 centre (122.1429, -36.2737) radius 2.25
  circle A806 centre (131.5714, -36.2737) radius 2.25
  circle A807 centre (141, -36.2737) radius 2.25
  circle A808 centre (150.4286, -36.2737) radius 2.25
  circle A809 centre (159.8571, -36.2737) radius 2.25
  circle A810 centre (169.2857, -36.2737) radius 2.25
  circle A811 centre (178.7143, -36.2737) radius 2.25
  circle A812 centre (188.1429, -36.2737) radius 2.25
  circle A813 centre (197.5714, -36.2737) radius 2.25
  circle A814 centre (207, -36.2737) radius 2.25
  circle A815 centre (216.4286, -36.2737) radius 2.25
  circle A816 centre (225.8571, -36.2737) radius 2.25
  circle A817 centre (235.2857, -36.2737) radius 2.25
  circle A818 centre (244.7143, -36.2737) radius 2.25
  circle A819 centre (254.1429, -36.2737) radius 2.25
  circle A820 centre (263.5714, -36.2737) radius 2.25
  circle A821 centre (273, -36.2737) radius 2.25
  circle A822 centre (282.4286, -36.2737) radius 2.25
  circle A823 centre (291.8571, -36.2737) radius 2.25
  circle A824 centre (301.2857, -36.2737) radius 2.25
  circle A825 centre (310.7143, -36.2737) radius 2.25
  circle A826 centre (320.1429, -36.2737) radius 2.25
  circle A827 centre (329.5714, -36.2737) radius 2.25
  circle A828 centre (339, -36.2737) radius 2.25
  circle A829 centre (348.4286, -36.2737) radius 2.25
  circle A830 centre (357.8571, -36.2737) radius 2.25
  circle A831 centre (367.2857, -36.2737) radius 2.25
  circle A832 centre (376.7143, -36.2737) radius 2.25
  circle A833 centre (386.1429, -36.2737) radius 2.25
  circle A834 centre (395.5714, -36.2737) radius 2.25
  circle A835 centre (405, -36.2737) radius 2.25
  circle A836 centre (75, -26.9158) radius 2.25
  circle A837 centre (84.4286, -26.9158) radius 2.25
  circle A838 centre (93.8571, -26.9158) radius 2.25
  circle A839 centre (103.2857, -26.9158) radius 2.25
  circle A840 centre (112.7143, -26.9158) radius 2.25
  circle A841 centre (122.1429, -26.9158) radius 2.25
  circle A842 centre (131.5714, -26.9158) radius 2.25
  circle A843 centre (141, -26.9158) radius 2.25
  circle A844 centre (150.4286, -26.9158) radius 2.25
  circle A845 centre (159.8571, -26.9158) radius 2.25
  circle A846 centre (169.2857, -26.9158) radius 2.25
  circle A847 centre (178.7143, -26.9158) radius 2.25
  circle A848 centre (188.1429, -26.9158) radius 2.25
  circle A849 centre (197.5714, -26.9158) radius 2.25
  circle A850 centre (207, -26.9158) radius 2.25
  circle A851 centre (216.4286, -26.9158) radius 2.25
  circle A852 centre (225.8571, -26.9158) radius 2.25
  circle A853 centre (235.2857, -26.9158) radius 2.25
  circle A854 centre (244.7143, -26.9158) radius 2.25
  circle A855 centre (254.1429, -26.9158) radius 2.25
  circle A856 centre (263.5714, -26.9158) radius 2.25
  circle A857 centre (273, -26.9158) radius 2.25
  circle A858 centre (282.4286, -26.9158) radius 2.25
  circle A859 centre (291.8571, -26.9158) radius 2.25
  circle A860 centre (301.2857, -26.9158) radius 2.25
  circle A861 centre (310.7143, -26.9158) radius 2.25
  circle A862 centre (320.1429, -26.9158) radius 2.25
  circle A863 centre (329.5714, -26.9158) radius 2.25
  circle A864 centre (339, -26.9158) radius 2.25
  circle A865 centre (348.4286, -26.9158) radius 2.25
  circle A866 centre (357.8571, -26.9158) radius 2.25
  circle A867 centre (367.2857, -26.9158) radius 2.25
  circle A868 centre (376.7143, -26.9158) radius 2.25
  circle A869 centre (386.1429, -26.9158) radius 2.25
  circle A870 centre (395.5714, -26.9158) radius 2.25
  circle A871 centre (405, -26.9158) radius 2.25
  circle A872 centre (75, -17.5579) radius 2.25
  circle A873 centre (84.4286, -17.5579) radius 2.25
  circle A874 centre (93.8571, -17.5579) radius 2.25
  circle A875 centre (103.2857, -17.5579) radius 2.25
  circle A876 centre (112.7143, -17.5579) radius 2.25
  circle A877 centre (122.1429, -17.5579) radius 2.25
  circle A878 centre (131.5714, -17.5579) radius 2.25
  circle A879 centre (141, -17.5579) radius 2.25
  circle A880 centre (150.4286, -17.5579) radius 2.25
  circle A881 centre (159.8571, -17.5579) radius 2.25
  circle A882 centre (169.2857, -17.5579) radius 2.25
  circle A883 centre (178.7143, -17.5579) radius 2.25
  circle A884 centre (188.1429, -17.5579) radius 2.25
  circle A885 centre (197.5714, -17.5579) radius 2.25
  circle A886 centre (207, -17.5579) radius 2.25
  circle A887 centre (216.4286, -17.5579) radius 2.25
  circle A888 centre (225.8571, -17.5579) radius 2.25
  circle A889 centre (235.2857, -17.5579) radius 2.25
  circle A890 centre (244.7143, -17.5579) radius 2.25
  circle A891 centre (254.1429, -17.5579) radius 2.25
  circle A892 centre (263.5714, -17.5579) radius 2.25
  circle A893 centre (273, -17.5579) radius 2.25
  circle A894 centre (282.4286, -17.5579) radius 2.25
  circle A895 centre (291.8571, -17.5579) radius 2.25
  circle A896 centre (301.2857, -17.5579) radius 2.25
  circle A897 centre (310.7143, -17.5579) radius 2.25
  circle A898 centre (320.1429, -17.5579) radius 2.25
  circle A899 centre (329.5714, -17.5579) radius 2.25
  circle A900 centre (339, -17.5579) radius 2.25
  circle A901 centre (348.4286, -17.5579) radius 2.25
  circle A902 centre (357.8571, -17.5579) radius 2.25
  circle A903 centre (367.2857, -17.5579) radius 2.25
  circle A904 centre (376.7143, -17.5579) radius 2.25
  circle A905 centre (386.1429, -17.5579) radius 2.25
  circle A906 centre (395.5714, -17.5579) radius 2.25
  circle A907 centre (405, -17.5579) radius 2.25
  circle A908 centre (75, -8.2) radius 2.25
  circle A909 centre (84.4286, -8.2) radius 2.25
  circle A910 centre (93.8571, -8.2) radius 2.25
  circle A911 centre (103.2857, -8.2) radius 2.25
  circle A912 centre (112.7143, -8.2) radius 2.25
  circle A913 centre (122.1429, -8.2) radius 2.25
  circle A914 centre (131.5714, -8.2) radius 2.25
  circle A915 centre (141, -8.2) radius 2.25
  circle A916 centre (150.4286, -8.2) radius 2.25
  circle A917 centre (159.8571, -8.2) radius 2.25
  circle A918 centre (169.2857, -8.2) radius 2.25
  circle A919 centre (178.7143, -8.2) radius 2.25
  circle A920 centre (188.1429, -8.2) radius 2.25
  circle A921 centre (197.5714, -8.2) radius 2.25
  circle A922 centre (207, -8.2) radius 2.25
  circle A923 centre (216.4286, -8.2) radius 2.25
  circle A924 centre (225.8571, -8.2) radius 2.25
  circle A925 centre (235.2857, -8.2) radius 2.25
  circle A926 centre (244.7143, -8.2) radius 2.25
  circle A927 centre (254.1429, -8.2) radius 2.25
  circle A928 centre (263.5714, -8.2) radius 2.25
  circle A929 centre (273, -8.2) radius 2.25
  circle A930 centre (282.4286, -8.2) radius 2.25
  circle A931 centre (291.8571, -8.2) radius 2.25